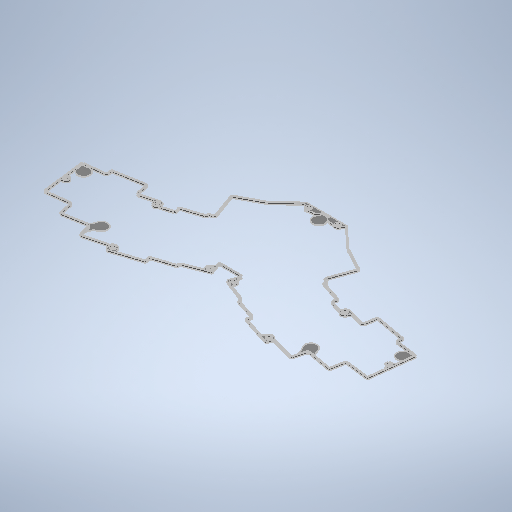
# Autodesk Inventor part: Hephaestus38v2 Case Bottom
Saved by Autodesk Inventor 2025 (Build 290162000, 162)
## iProperties
Created: 2025-11-22
Part Number: Hephaestus38v2 Case Bottom
Material: Generic
Document SubType Name: Modeling
Designer: User
Density: 1 g/cm^3
Appearance: Smooth - Black
Author: User
Autodesk Inventor part; units mm, degrees
(part 1 of 2)
ref_plane "YZ Plane" through (0, 0, 0) normal (1, 0, 0) x (0, 1, 0)
ref_plane "XZ Plane" through (0, 0, 0) normal (0, 1, 0) x (-1, 0, 0)
ref_plane "XY Plane" through (0, 0, 0) normal (0, 0, 1) x (1, 0, 0)
sketch "Sketch1" plane through (0, 0, 0) normal (0, 1, 0) x (-1, 0, 0)
  line L0 (-4.3858, 37.0574) -> (-22.4739, 44.0008)
  circle A0 centre (-7.0476, 34.7035) radius 1.1
  arc A1 (9.4036, 37.0574) -> (8.8284, 35.7654) centre (9.762, 36.1238) ccw
  line L1 (8.8284, 35.7654) -> (11.5745, 28.6116)
  arc A2 (10.6409, 27.2532) -> (11.5745, 28.6116) centre (10.641, 28.2531) ccw
  line L2 (10.6409, 27.2532) -> (-5.6231, 27.2532)
  arc A3 (-6.5567, 28.6116) -> (-5.6231, 27.2532) centre (-5.623, 28.2533) ccw
  line L3 (-6.5567, 28.6116) -> (-3.8105, 35.7654)
  arc A4 (-3.8105, 35.7654) -> (-4.3858, 37.0574) centre (-4.744, 36.1239) ccw
  line L4 (-4.3858, 37.0574) -> (-22.4739, 44.0008)
  arc A5 (-23.0666, 45.2434) -> (-22.4739, 44.0008) centre (-22.1155, 44.9344) ccw
  line L5 (-23.0666, 45.2434) -> (-22.9423, 45.6258)
  arc A6 (-22.9423, 45.6258) -> (-23.5844, 46.8859) centre (-23.8933, 45.9349) ccw
  circle A7 centre (12.0655, 34.7035) radius 1.1
  line L6 (10.6409, 27.2532) -> (-5.6231, 27.2532)
  arc A8 (10.6409, 27.2532) -> (11.5745, 28.6116) centre (10.641, 28.2531) ccw
  line L7 (-6.5567, 28.6116) -> (-3.8105, 35.7654)
  arc A9 (-3.8105, 35.7654) -> (-4.3858, 37.0574) centre (-4.744, 36.1239) ccw
  line L8 (8.8284, 35.7654) -> (11.5745, 28.6116)
  line L9 (27.4917, 44.0008) -> (9.4036, 37.0574)
  arc A10 (27.4917, 44.0008) -> (28.0844, 45.2433) centre (27.1334, 44.9343) ccw
  line L10 (27.9602, 45.6258) -> (28.0844, 45.2433)
  arc A11 (28.6022, 46.8859) -> (27.9602, 45.6258) centre (28.9113, 45.9348) ccw
  line L11 (44.7702, 52.1391) -> (28.6022, 46.8859)
  arc A12 (9.4036, 37.0574) -> (8.8284, 35.7654) centre (9.762, 36.1238) ccw
  arc A13 (45.2817, 57.0369) -> (44.6397, 55.7769) centre (45.5908, 56.0858) ccw
  line L12 (44.6397, 55.7769) -> (45.4122, 53.3992)
  arc A14 (44.7702, 52.1391) -> (45.4122, 53.3992) centre (44.4612, 53.0901) ccw
  line L13 (44.7702, 52.1391) -> (28.6022, 46.8859)
  arc A15 (28.6022, 46.8859) -> (27.9602, 45.6258) centre (28.9113, 45.9348) ccw
  line L14 (27.9602, 45.6258) -> (28.0844, 45.2433)
  arc A16 (27.4917, 44.0008) -> (28.0844, 45.2433) centre (27.1334, 44.9343) ccw
  line L15 (27.4917, 44.0008) -> (9.4036, 37.0574)
  line L16 (-23.5844, 46.8859) -> (-39.7523, 52.1392)
  arc A17 (-40.3944, 53.3993) -> (-39.7523, 52.1392) centre (-39.4433, 53.0903) ccw
  line L17 (-40.3944, 53.3993) -> (-39.6218, 55.7769)
  arc A18 (-39.6218, 55.7769) -> (-40.2638, 57.037) centre (-40.5728, 56.086) ccw
  circle A19 centre (-63.5707, 60.8956) radius 1.1
  circle A20 centre (68.5886, 60.8955) radius 1.1
  line L18 (20.0076, -53.7302) -> (36.7848, -38.2361)
  circle A21 centre (14.7393, -51.2055) radius 1.1
  arc A22 (-14.9899, -53.7302) -> (-14.3114, -53.9956) centre (-14.3114, -52.9955) ccw
  line L19 (-14.3114, -53.9956) -> (19.3291, -53.9956)
  line L20 (56.4521, -26.7701) -> (49.3032, -6.9462)
  arc A23 (36.9938, -38.0878) -> (36.7848, -38.2361) centre (37.4628, -38.97) ccw
  arc A24 (19.3291, -53.9956) -> (20.0076, -53.7302) centre (19.3291, -52.9954) ccw
  line L21 (20.0076, -53.7302) -> (36.7848, -38.2361)
  line L22 (36.9938, -38.0878) -> (55.9808, -27.9922)
  arc A25 (55.9808, -27.9922) -> (56.4521, -26.7701) centre (55.5114, -27.1093) ccw
  arc A26 (36.9938, -38.0878) -> (36.7848, -38.2361) centre (37.4628, -38.97) ccw
  line L23 (36.9938, -38.0878) -> (55.9808, -27.9922)
  arc A27 (55.9808, -27.9922) -> (56.4521, -26.7701) centre (55.5114, -27.1093) ccw
  line L24 (56.4521, -26.7701) -> (49.3032, -6.9462)
  arc A28 (53.4637, -2.2357) -> (52.8392, -3.5451) centre (53.7728, -3.1867) ccw
  line L25 (53.1719, -4.4119) -> (52.8392, -3.5451)
  line L26 (49.8855, -5.6734) -> (53.1719, -4.4119)
  arc A29 (69.7006, 7.7716) -> (69.0586, 6.5115) centre (70.0096, 6.8206) ccw
  line L27 (69.8311, 4.1339) -> (69.0586, 6.5115)
  arc A30 (69.1891, 2.8738) -> (69.8311, 4.1339) centre (68.8803, 3.8248) ccw
  line L28 (53.4637, -2.2357) -> (69.1891, 2.8738)
  line L29 (69.7006, 7.7716) -> (77.7078, 10.3732)
  arc A31 (78.9827, 9.681) -> (77.7078, 10.3732) centre (78.0168, 9.4221) ccw
  arc A32 (49.8855, -5.6734) -> (49.3032, -6.9462) centre (50.2437, -6.6069) ccw
  circle A33 centre (-76.6637, 9.8152) radius 1.1
  circle A34 centre (-133.8477, 29.6046) radius 1.1
  circle A35 centre (138.8656, 29.6043) radius 1.1
  circle A36 centre (81.6815, 9.8151) radius 1.1
  circle A37 centre (12.0655, 34.7035) radius 1.1
  circle A38 centre (-9.7216, -51.2055) radius 1.1
  circle A39 centre (-9.7216, -51.2055) radius 1.1
  circle A40 centre (14.7393, -51.2055) radius 1.1
  line L30 (-14.3114, -53.9956) -> (19.3291, -53.9956)
  arc A41 (-14.9899, -53.7302) -> (-14.3114, -53.9956) centre (-14.3114, -52.9955) ccw
  line L31 (-31.7671, -38.236) -> (-14.9899, -53.7302)
  arc A42 (19.3291, -53.9956) -> (20.0076, -53.7302) centre (19.3291, -52.9954) ccw
  arc A43 (-31.7671, -38.236) -> (-31.9761, -38.0877) centre (-32.4462, -38.9715) ccw
  line L32 (-50.9631, -27.9922) -> (-31.9761, -38.0877)
  arc A44 (-44.2854, -6.9461) -> (-44.8677, -5.6733) centre (-45.2262, -6.6069) ccw
  arc A45 (-51.4343, -26.77) -> (-50.9631, -27.9922) centre (-50.4936, -27.1092) ccw
  line L33 (-44.2854, -6.9461) -> (-51.4343, -26.77)
  line L34 (-47.2205, -4.7701) -> (-44.8677, -5.6733)
  arc A46 (-47.7958, -3.4782) -> (-47.2205, -4.7701) centre (-46.8621, -3.8365) ccw
  line L35 (-47.4437, -2.5612) -> (-47.7958, -3.4782)
  line L36 (-64.1713, 2.8739) -> (-47.4437, -2.5612)
  line L37 (-64.0408, 6.5116) -> (-64.8134, 4.134)
  arc A47 (-64.0408, 6.5116) -> (-64.6829, 7.7717) centre (-64.9919, 6.8206) ccw
  arc A48 (-64.8134, 4.134) -> (-64.1713, 2.8739) centre (-63.8622, 3.825) ccw
  line L38 (-72.69, 10.3734) -> (-64.6829, 7.7717)
  arc A49 (-75.8938, 6.3463) -> (-74.669, 7.0534) centre (-75.635, 7.3122) ccw
  line L39 (-74.669, 7.0534) -> (-73.9649, 9.6812)
  arc A50 (-72.69, 10.3734) -> (-73.9649, 9.6812) centre (-72.999, 9.4222) ccw
  line L40 (-111.7079, 56.9853) -> (-113.4989, 46.8282)
  line L41 (-120.3501, 7.9735) -> (-120.8071, 5.3814)
  arc A51 (-120.3501, 7.9735) -> (-121.213, 9.1397) centre (-121.3349, 8.1472) ccw
  line L42 (-137.7648, 11.1721) -> (-121.213, 9.1397)
  arc A52 (-133.2069, 48.2933) -> (-134.3213, 47.4226) centre (-133.3287, 47.3007) ccw
  line L43 (-134.3213, 47.4226) -> (-138.6355, 12.2865)
  arc A53 (-138.6355, 12.2865) -> (-137.7648, 11.1721) centre (-137.6431, 12.1645) ccw
  arc A54 (-90.8984, 54.3314) -> (-89.7588, 55.0574) centre (-90.7247, 55.3162) ccw
  arc A55 (-114.6056, 46.0093) -> (-113.4989, 46.8282) centre (-114.4838, 47.0019) ccw
  arc A56 (-110.5495, 57.7965) -> (-111.7079, 56.9853) centre (-110.7232, 56.8118) ccw
  line L44 (-114.6056, 46.0093) -> (-133.2069, 48.2933)
  line L45 (-90.8984, 54.3314) -> (-110.5495, 57.7965)
  line L46 (-40.2638, 57.037) -> (-64.0403, 64.7624)
  circle A57 centre (-63.5707, 60.8956) radius 1.1
  arc A58 (-67.5003, 60.4163) -> (-66.2904, 61.0732) centre (-67.2415, 61.3823) ccw
  arc A59 (-64.0403, 64.7624) -> (-65.3003, 64.1204) centre (-64.3492, 63.8113) ccw
  line L47 (-65.3003, 64.1204) -> (-66.2904, 61.0732)
  line L48 (-91.3846, 10.4971) -> (-75.8938, 6.3463)
  arc A60 (-95.3758, -0.1183) -> (-94.2173, 0.6929) centre (-95.2021, 0.8665) ccw
  arc A61 (-91.3846, 10.4971) -> (-92.6283, 9.7048) centre (-91.6435, 9.5312) ccw
  line L49 (-94.2173, 0.6929) -> (-92.6283, 9.7048)
  arc A62 (-120.8071, 5.3814) -> (-119.996, 4.2229) centre (-119.8224, 5.2077) ccw
  line L50 (-119.996, 4.2229) -> (-95.3758, -0.1183)
  arc A63 (69.7006, 7.7716) -> (69.0586, 6.5115) centre (70.0096, 6.8206) ccw
  arc A64 (53.4637, -2.2357) -> (52.8392, -3.5451) centre (53.7728, -3.1867) ccw
  line L51 (53.1719, -4.4119) -> (52.8392, -3.5451)
  line L52 (49.8855, -5.6734) -> (53.1719, -4.4119)
  line L53 (69.8311, 4.1339) -> (69.0586, 6.5115)
  arc A65 (69.1891, 2.8738) -> (69.8311, 4.1339) centre (68.8803, 3.8248) ccw
  line L54 (53.4637, -2.2357) -> (69.1891, 2.8738)
  line L55 (69.7006, 7.7716) -> (77.7078, 10.3732)
  arc A66 (49.8855, -5.6734) -> (49.3032, -6.9462) centre (50.2437, -6.6069) ccw
  line L56 (69.0581, 64.7623) -> (45.2817, 57.0369)
  arc A67 (70.3182, 64.1203) -> (69.0581, 64.7623) centre (69.3671, 63.8112) ccw
  arc A68 (71.3083, 61.0731) -> (72.5182, 60.4162) centre (72.2593, 61.3821) ccw
  line L57 (90.98, 65.363) -> (72.5182, 60.4162)
  arc A69 (92.2048, 64.6558) -> (90.98, 65.363) centre (91.2388, 64.397) ccw
  arc A70 (94.7767, 55.0573) -> (95.9163, 54.3313) centre (95.7426, 55.3161) ccw
  line L58 (94.7767, 55.0573) -> (92.2048, 64.6558)
  line L59 (71.3083, 61.0731) -> (70.3182, 64.1203)
  arc A71 (142.7826, 11.1718) -> (143.6533, 12.2863) centre (142.6606, 12.1645) ccw
  line L60 (78.9827, 9.681) -> (79.6868, 7.0532)
  arc A72 (79.6868, 7.0532) -> (80.9116, 6.3461) centre (80.6528, 7.3122) ccw
  line L61 (80.9116, 6.3461) -> (96.4024, 10.4969)
  arc A73 (97.6461, 9.7046) -> (96.4024, 10.4969) centre (96.6613, 9.531) ccw
  line L62 (97.6461, 9.7046) -> (99.2351, 0.6927)
  arc A74 (99.2351, 0.6927) -> (100.3935, -0.1185) centre (100.2199, 0.8664) ccw
  line L63 (100.3935, -0.1185) -> (125.0138, 4.2228)
  arc A75 (126.2308, 9.1395) -> (125.3678, 7.9733) centre (126.3526, 8.147) ccw
  arc A76 (125.0138, 4.2228) -> (125.8249, 5.3812) centre (124.8401, 5.2075) ccw
  line L64 (125.8249, 5.3812) -> (125.3678, 7.9733)
  line L65 (115.5673, 57.7963) -> (95.9163, 54.3313)
  arc A77 (116.7258, 56.9851) -> (115.5673, 57.7963) centre (115.7409, 56.8114) ccw
  line L66 (118.5167, 46.828) -> (116.7258, 56.9851)
  arc A78 (118.5167, 46.828) -> (119.6234, 46.0091) centre (119.5015, 47.0016) ccw
  arc A79 (139.3392, 47.4224) -> (138.2247, 48.2931) centre (138.3466, 47.3005) ccw
  line L67 (126.2308, 9.1395) -> (142.7826, 11.1718)
  line L68 (143.6533, 12.2863) -> (139.3392, 47.4224)
  arc A80 (142.7826, 11.1718) -> (143.6533, 12.2863) centre (142.6606, 12.1645) ccw
  line L69 (138.2247, 48.2931) -> (119.6234, 46.0091)
  circle A81 centre (68.5886, 60.8955) radius 1.1
  circle A82 centre (-7.0476, 34.7035) radius 1.1
  arc A83 (-31.7671, -38.236) -> (-31.9761, -38.0877) centre (-32.4462, -38.9715) ccw
  line L70 (-50.9631, -27.9922) -> (-31.9761, -38.0877)
  arc A84 (-51.4343, -26.77) -> (-50.9631, -27.9922) centre (-50.4936, -27.1092) ccw
  line L71 (-44.2854, -6.9461) -> (-51.4343, -26.77)
  arc A85 (-44.2854, -6.9461) -> (-44.8677, -5.6733) centre (-45.2262, -6.6069) ccw
  line L72 (-47.2205, -4.7701) -> (-44.8677, -5.6733)
  arc A86 (-47.7958, -3.4782) -> (-47.2205, -4.7701) centre (-46.8621, -3.8365) ccw
  line L73 (-47.4437, -2.5612) -> (-47.7958, -3.4782)
  circle A87 centre (-133.8477, 29.6046) radius 1.1
  line L74 (-31.7671, -38.236) -> (-14.9899, -53.7302)
  circle A88 centre (-76.6637, 9.8152) radius 1.1
  line L75 (-23.0666, 45.2434) -> (-22.9423, 45.6258)
  arc A89 (-23.0666, 45.2434) -> (-22.4739, 44.0008) centre (-22.1155, 44.9344) ccw
  arc A90 (-22.9423, 45.6258) -> (-23.5844, 46.8859) centre (-23.8933, 45.9349) ccw
  line L76 (-23.5844, 46.8859) -> (-39.7523, 52.1392)
  arc A91 (-39.6218, 55.7769) -> (-40.2638, 57.037) centre (-40.5728, 56.086) ccw
  line L77 (-40.3944, 53.3993) -> (-39.6218, 55.7769)
  arc A92 (-40.3944, 53.3993) -> (-39.7523, 52.1392) centre (-39.4433, 53.0903) ccw
  arc A93 (-6.5567, 28.6116) -> (-5.6231, 27.2532) centre (-5.623, 28.2533) ccw
  line L78 (-40.2638, 57.037) -> (-64.0403, 64.7624)
  arc A94 (-64.0403, 64.7624) -> (-65.3003, 64.1204) centre (-64.3492, 63.8113) ccw
  line L79 (-65.3003, 64.1204) -> (-66.2904, 61.0732)
  arc A95 (-67.5003, 60.4163) -> (-66.2904, 61.0732) centre (-67.2415, 61.3823) ccw
  arc A96 (94.7767, 55.0573) -> (95.9163, 54.3313) centre (95.7426, 55.3161) ccw
  circle A97 centre (81.6815, 9.8151) radius 1.1
  line L80 (100.3935, -0.1185) -> (125.0138, 4.2228)
  arc A98 (125.0138, 4.2228) -> (125.8249, 5.3812) centre (124.8401, 5.2075) ccw
  arc A99 (99.2351, 0.6927) -> (100.3935, -0.1185) centre (100.2199, 0.8664) ccw
  arc A100 (78.9827, 9.681) -> (77.7078, 10.3732) centre (78.0168, 9.4221) ccw
  line L81 (78.9827, 9.681) -> (79.6868, 7.0532)
  arc A101 (79.6868, 7.0532) -> (80.9116, 6.3461) centre (80.6528, 7.3122) ccw
  line L82 (80.9116, 6.3461) -> (96.4024, 10.4969)
  arc A102 (97.6461, 9.7046) -> (96.4024, 10.4969) centre (96.6613, 9.531) ccw
  line L83 (125.8249, 5.3812) -> (125.3678, 7.9733)
  arc A103 (126.2308, 9.1395) -> (125.3678, 7.9733) centre (126.3526, 8.147) ccw
  line L84 (97.6461, 9.7046) -> (99.2351, 0.6927)
  circle A104 centre (138.8656, 29.6043) radius 1.1
  arc A105 (118.5167, 46.828) -> (119.6234, 46.0091) centre (119.5015, 47.0016) ccw
  line L85 (138.2247, 48.2931) -> (119.6234, 46.0091)
  line L86 (126.2308, 9.1395) -> (142.7826, 11.1718)
  arc A106 (139.3392, 47.4224) -> (138.2247, 48.2931) centre (138.3466, 47.3005) ccw
  line L87 (143.6533, 12.2863) -> (139.3392, 47.4224)
  arc A107 (71.3083, 61.0731) -> (72.5182, 60.4162) centre (72.2593, 61.3821) ccw
  line L88 (90.98, 65.363) -> (72.5182, 60.4162)
  arc A108 (92.2048, 64.6558) -> (90.98, 65.363) centre (91.2388, 64.397) ccw
  line L89 (94.7767, 55.0573) -> (92.2048, 64.6558)
  line L90 (115.5673, 57.7963) -> (95.9163, 54.3313)
  arc A109 (116.7258, 56.9851) -> (115.5673, 57.7963) centre (115.7409, 56.8114) ccw
  line L91 (118.5167, 46.828) -> (116.7258, 56.9851)
  arc A110 (44.7702, 52.1391) -> (45.4122, 53.3992) centre (44.4612, 53.0901) ccw
  line L92 (44.6397, 55.7769) -> (45.4122, 53.3992)
  arc A111 (45.2817, 57.0369) -> (44.6397, 55.7769) centre (45.5908, 56.0858) ccw
  line L93 (69.0581, 64.7623) -> (45.2817, 57.0369)
  line L94 (71.3083, 61.0731) -> (70.3182, 64.1203)
  arc A112 (70.3182, 64.1203) -> (69.0581, 64.7623) centre (69.3671, 63.8112) ccw
  line L95 (-72.69, 10.3734) -> (-64.6829, 7.7717)
  arc A113 (-72.69, 10.3734) -> (-73.9649, 9.6812) centre (-72.999, 9.4222) ccw
  line L96 (-74.669, 7.0534) -> (-73.9649, 9.6812)
  arc A114 (-75.8938, 6.3463) -> (-74.669, 7.0534) centre (-75.635, 7.3122) ccw
  line L97 (-91.3846, 10.4971) -> (-75.8938, 6.3463)
  arc A115 (-91.3846, 10.4971) -> (-92.6283, 9.7048) centre (-91.6435, 9.5312) ccw
  line L98 (-94.2173, 0.6929) -> (-92.6283, 9.7048)
  arc A116 (-138.6355, 12.2865) -> (-137.7648, 11.1721) centre (-137.6431, 12.1645) ccw
  line L99 (-137.7648, 11.1721) -> (-121.213, 9.1397)
  arc A117 (-120.3501, 7.9735) -> (-121.213, 9.1397) centre (-121.3349, 8.1472) ccw
  line L100 (-120.3501, 7.9735) -> (-120.8071, 5.3814)
  arc A118 (-120.8071, 5.3814) -> (-119.996, 4.2229) centre (-119.8224, 5.2077) ccw
  line L101 (-119.996, 4.2229) -> (-95.3758, -0.1183)
  arc A119 (-133.2069, 48.2933) -> (-134.3213, 47.4226) centre (-133.3287, 47.3007) ccw
  arc A120 (-114.6056, 46.0093) -> (-113.4989, 46.8282) centre (-114.4838, 47.0019) ccw
  line L102 (-114.6056, 46.0093) -> (-133.2069, 48.2933)
  line L103 (-67.5003, 60.4163) -> (-85.9621, 65.3631)
  line L104 (-67.5003, 60.4163) -> (-85.9621, 65.3631)
  line L105 (-64.1713, 2.8739) -> (-47.4437, -2.5612)
  arc A121 (-64.8134, 4.134) -> (-64.1713, 2.8739) centre (-63.8622, 3.825) ccw
  line L106 (-64.0408, 6.5116) -> (-64.8134, 4.134)
  arc A122 (-64.0408, 6.5116) -> (-64.6829, 7.7717) centre (-64.9919, 6.8206) ccw
  arc A123 (-95.3758, -0.1183) -> (-94.2173, 0.6929) centre (-95.2021, 0.8665) ccw
  line L107 (-90.8984, 54.3314) -> (-110.5495, 57.7965)
  line L108 (-111.7079, 56.9853) -> (-113.4989, 46.8282)
  arc A124 (-85.9621, 65.3631) -> (-87.1869, 64.656) centre (-86.2209, 64.3972) ccw
  arc A125 (-85.9621, 65.3631) -> (-87.1869, 64.656) centre (-86.2209, 64.3972) ccw
  line L109 (-87.1869, 64.656) -> (-89.7588, 55.0574)
  line L110 (-87.1869, 64.656) -> (-89.7588, 55.0574)
  arc A126 (-90.8984, 54.3314) -> (-89.7588, 55.0574) centre (-90.7247, 55.3162) ccw
  arc A127 (-110.5495, 57.7965) -> (-111.7079, 56.9853) centre (-110.7232, 56.8118) ccw
  line L111 (-134.3213, 47.4226) -> (-138.6355, 12.2865)
  constraints: 224 end point, 216 point on circle, 128 centre point, 2 horizontal, 476 other
extrude "Extrusion1" add sketch "Sketch1" along normal blind 1.6
sketch "Sketch2" plane through (0, 1.6, 0) normal (0, 1, 0) x (1, 0, 0)
  arc A0 (90.8984, -54.3314) -> (89.7588, -55.0574) centre (90.7247, -55.3162) ccw projected
  line L0 (90.8984, -54.3314) -> (110.5495, -57.7965) projected
  arc A1 (110.5495, -57.7965) -> (111.7079, -56.9853) centre (110.7232, -56.8118) ccw projected
  line L1 (111.7079, -56.9853) -> (113.4989, -46.8282) projected
  arc A2 (114.6056, -46.0093) -> (113.4989, -46.8282) centre (114.4838, -47.0019) ccw projected
  line L2 (114.6056, -46.0093) -> (133.2069, -48.2933) projected
  arc A3 (133.2069, -48.2933) -> (134.3213, -47.4226) centre (133.3287, -47.3007) ccw projected
  line L3 (134.3213, -47.4226) -> (138.6355, -12.2865) projected
  arc A4 (138.6355, -12.2865) -> (137.7648, -11.1721) centre (137.6431, -12.1645) ccw projected
  line L4 (137.7648, -11.1721) -> (121.213, -9.1397) projected
  arc A5 (120.3501, -7.9735) -> (121.213, -9.1397) centre (121.3349, -8.1472) ccw projected
  line L5 (120.3501, -7.9735) -> (120.8071, -5.3814) projected
  arc A6 (120.8071, -5.3814) -> (119.996, -4.2229) centre (119.8224, -5.2077) ccw projected
  line L6 (119.996, -4.2229) -> (95.3758, 0.1183) projected
  arc A7 (95.3758, 0.1183) -> (94.2173, -0.6929) centre (95.2021, -0.8665) ccw projected
  line L7 (94.2173, -0.6929) -> (92.6283, -9.7048) projected
  arc A8 (91.3846, -10.4971) -> (92.6283, -9.7048) centre (91.6435, -9.5312) ccw projected
  line L8 (91.3846, -10.4971) -> (75.8938, -6.3463) projected
  arc A9 (75.8938, -6.3463) -> (74.669, -7.0534) centre (75.635, -7.3122) ccw projected
  line L9 (74.669, -7.0534) -> (73.9649, -9.6812) projected
  arc A10 (72.69, -10.3734) -> (73.9649, -9.6812) centre (72.999, -9.4222) ccw projected
  line L10 (72.69, -10.3734) -> (64.6829, -7.7717) projected
  arc A11 (64.0408, -6.5116) -> (64.6829, -7.7717) centre (64.9919, -6.8206) ccw projected
  line L11 (64.0408, -6.5116) -> (64.8134, -4.134) projected
  arc A12 (64.8134, -4.134) -> (64.1713, -2.8739) centre (63.8622, -3.825) ccw projected
  line L12 (64.1713, -2.8739) -> (47.4437, 2.5612) projected
  line L13 (47.4437, 2.5612) -> (47.7958, 3.4782) projected
  arc A13 (47.7958, 3.4782) -> (47.2205, 4.7701) centre (46.8621, 3.8365) ccw projected
  line L14 (47.2205, 4.7701) -> (44.8677, 5.6733) projected
  arc A14 (44.2854, 6.9461) -> (44.8677, 5.6733) centre (45.2262, 6.6069) ccw projected
  line L15 (44.2854, 6.9461) -> (51.4343, 26.77) projected
  arc A15 (51.4343, 26.77) -> (50.9631, 27.9922) centre (50.4936, 27.1092) ccw projected
  line L16 (50.9631, 27.9922) -> (31.9761, 38.0877) projected
  arc A16 (31.7671, 38.236) -> (31.9761, 38.0877) centre (32.4462, 38.9715) ccw projected
  line L17 (31.7671, 38.236) -> (14.9899, 53.7302) projected
  arc A17 (14.9899, 53.7302) -> (14.3114, 53.9956) centre (14.3114, 52.9955) ccw projected
  line L18 (14.3114, 53.9956) -> (-19.3291, 53.9956) projected
  arc A18 (-19.3291, 53.9956) -> (-20.0076, 53.7302) centre (-19.3291, 52.9954) ccw projected
  line L19 (-20.0076, 53.7302) -> (-36.7848, 38.2361) projected
  arc A19 (-36.9938, 38.0878) -> (-36.7848, 38.2361) centre (-37.4628, 38.97) ccw projected
  line L20 (-36.9938, 38.0878) -> (-55.9808, 27.9922) projected
  arc A20 (-55.9808, 27.9922) -> (-56.4521, 26.7701) centre (-55.5114, 27.1093) ccw projected
  line L21 (-56.4521, 26.7701) -> (-49.3032, 6.9462) projected
  arc A21 (-49.8855, 5.6734) -> (-49.3032, 6.9462) centre (-50.2437, 6.6069) ccw projected
  line L22 (-49.8855, 5.6734) -> (-53.1719, 4.4119) projected
  line L23 (-53.1719, 4.4119) -> (-52.8392, 3.5451) projected
  arc A22 (-53.4637, 2.2357) -> (-52.8392, 3.5451) centre (-53.7728, 3.1867) ccw projected
  line L24 (-53.4637, 2.2357) -> (-69.1891, -2.8738) projected
  arc A23 (-69.1891, -2.8738) -> (-69.8311, -4.1339) centre (-68.8803, -3.8248) ccw projected
  line L25 (-69.8311, -4.1339) -> (-69.0586, -6.5115) projected
  arc A24 (-69.7006, -7.7716) -> (-69.0586, -6.5115) centre (-70.0096, -6.8206) ccw projected
  line L26 (-69.7006, -7.7716) -> (-77.7078, -10.3732) projected
  arc A25 (-78.9827, -9.681) -> (-77.7078, -10.3732) centre (-78.0168, -9.4221) ccw projected
  line L27 (-78.9827, -9.681) -> (-79.6868, -7.0532) projected
  arc A26 (-79.6868, -7.0532) -> (-80.9116, -6.3461) centre (-80.6528, -7.3122) ccw projected
  line L28 (-80.9116, -6.3461) -> (-96.4024, -10.4969) projected
  arc A27 (-97.6461, -9.7046) -> (-96.4024, -10.4969) centre (-96.6613, -9.531) ccw projected
  line L29 (-97.6461, -9.7046) -> (-99.2351, -0.6927) projected
  arc A28 (-99.2351, -0.6927) -> (-100.3935, 0.1185) centre (-100.2199, -0.8664) ccw projected
  line L30 (-100.3935, 0.1185) -> (-125.0138, -4.2228) projected
  arc A29 (-125.0138, -4.2228) -> (-125.8249, -5.3812) centre (-124.8401, -5.2075) ccw projected
  line L31 (-125.8249, -5.3812) -> (-125.3678, -7.9733) projected
  arc A30 (-126.2308, -9.1395) -> (-125.3678, -7.9733) centre (-126.3526, -8.147) ccw projected
  line L32 (-126.2308, -9.1395) -> (-142.7826, -11.1718) projected
  arc A31 (-142.7826, -11.1718) -> (-143.6533, -12.2863) centre (-142.6606, -12.1645) ccw projected
  line L33 (-143.6533, -12.2863) -> (-139.3392, -47.4224) projected
  arc A32 (-139.3392, -47.4224) -> (-138.2247, -48.2931) centre (-138.3466, -47.3005) ccw projected
  line L34 (-138.2247, -48.2931) -> (-119.6234, -46.0091) projected
  arc A33 (-118.5167, -46.828) -> (-119.6234, -46.0091) centre (-119.5015, -47.0016) ccw projected
  line L35 (-118.5167, -46.828) -> (-116.7258, -56.9851) projected
  arc A34 (-116.7258, -56.9851) -> (-115.5673, -57.7963) centre (-115.7409, -56.8114) ccw projected
  line L36 (-115.5673, -57.7963) -> (-95.9163, -54.3313) projected
  arc A35 (-94.7767, -55.0573) -> (-95.9163, -54.3313) centre (-95.7426, -55.3161) ccw projected
  line L37 (-94.7767, -55.0573) -> (-92.2048, -64.6558) projected
  arc A36 (-92.2048, -64.6558) -> (-90.98, -65.363) centre (-91.2388, -64.397) ccw projected
  line L38 (-90.98, -65.363) -> (-72.5182, -60.4162) projected
  arc A37 (-71.3083, -61.0731) -> (-72.5182, -60.4162) centre (-72.2593, -61.3821) ccw projected
  line L39 (-71.3083, -61.0731) -> (-70.3182, -64.1203) projected
  arc A38 (-70.3182, -64.1203) -> (-69.0581, -64.7623) centre (-69.3671, -63.8112) ccw projected
  line L40 (-69.0581, -64.7623) -> (-45.2817, -57.0369) projected
  arc A39 (-45.2817, -57.0369) -> (-44.6397, -55.7769) centre (-45.5908, -56.0858) ccw projected
  line L41 (-44.6397, -55.7769) -> (-45.4122, -53.3992) projected
  arc A40 (-44.7702, -52.1391) -> (-45.4122, -53.3992) centre (-44.4612, -53.0901) ccw projected
  line L42 (-44.7702, -52.1391) -> (-28.6022, -46.8859) projected
  arc A41 (-28.6022, -46.8859) -> (-27.9602, -45.6258) centre (-28.9113, -45.9348) ccw projected
  line L43 (-27.9602, -45.6258) -> (-28.0844, -45.2433) projected
  arc A42 (-27.4917, -44.0008) -> (-28.0844, -45.2433) centre (-27.1334, -44.9343) ccw projected
  line L44 (-27.4917, -44.0008) -> (-9.4036, -37.0574) projected
  arc A43 (-9.4036, -37.0574) -> (-8.8284, -35.7654) centre (-9.762, -36.1238) ccw projected
  line L45 (-8.8284, -35.7654) -> (-11.5745, -28.6116) projected
  arc A44 (-10.6409, -27.2532) -> (-11.5745, -28.6116) centre (-10.641, -28.2531) ccw projected
  line L46 (-10.6409, -27.2532) -> (5.6231, -27.2532) projected
  arc A45 (6.5567, -28.6116) -> (5.6231, -27.2532) centre (5.623, -28.2533) ccw projected
  line L47 (6.5567, -28.6116) -> (3.8105, -35.7654) projected
  arc A46 (3.8105, -35.7654) -> (4.3858, -37.0574) centre (4.744, -36.1239) ccw projected
  line L48 (4.3858, -37.0574) -> (22.4739, -44.0008) projected
  arc A47 (23.0666, -45.2434) -> (22.4739, -44.0008) centre (22.1155, -44.9344) ccw projected
  line L49 (23.0666, -45.2434) -> (22.9423, -45.6258) projected
  arc A48 (22.9423, -45.6258) -> (23.5844, -46.8859) centre (23.8933, -45.9349) ccw projected
  line L50 (23.5844, -46.8859) -> (39.7523, -52.1392) projected
  arc A49 (40.3944, -53.3993) -> (39.7523, -52.1392) centre (39.4433, -53.0903) ccw projected
  line L51 (40.3944, -53.3993) -> (39.6218, -55.7769) projected
  arc A50 (39.6218, -55.7769) -> (40.2638, -57.037) centre (40.5728, -56.086) ccw projected
  line L52 (40.2638, -57.037) -> (64.0403, -64.7624) projected
  arc A51 (64.0403, -64.7624) -> (65.3003, -64.1204) centre (64.3492, -63.8113) ccw projected
  line L53 (65.3003, -64.1204) -> (66.2904, -61.0732) projected
  arc A52 (67.5003, -60.4163) -> (66.2904, -61.0732) centre (67.2415, -61.3823) ccw projected
  line L54 (67.5003, -60.4163) -> (85.9621, -65.3631) projected
  arc A53 (85.9621, -65.3631) -> (87.1869, -64.656) centre (86.2209, -64.3972) ccw projected
  line L55 (87.1869, -64.656) -> (89.7588, -55.0574) projected
  circle A54 centre (9.7216, 51.2055) radius 1.1 projected
  circle A55 centre (-138.8656, -29.6043) radius 1.1 projected
  circle A56 centre (76.6637, -9.8152) radius 1.1 projected
  circle A57 centre (-14.7393, 51.2055) radius 1.1 projected
  circle A58 centre (-68.5886, -60.8955) radius 1.1 projected
  circle A59 centre (63.5707, -60.8956) radius 1.1 projected
  circle A60 centre (-12.0655, -34.7035) radius 1.1 projected
  circle A61 centre (7.0476, -34.7035) radius 1.1 projected
  circle A62 centre (133.8477, -29.6046) radius 1.1 projected
  circle A63 centre (-81.6815, -9.8151) radius 1.1 projected
  circle A64 centre (-14.7393, 51.2055) radius 2.25
  circle A65 centre (9.7216, 51.2055) radius 2.25
  circle A66 centre (76.6637, -9.8152) radius 2.25
  circle A67 centre (133.8477, -29.6046) radius 2.25
  circle A68 centre (63.5707, -60.8956) radius 2.25
  circle A69 centre (7.0476, -34.7035) radius 2.25
  circle A70 centre (-12.0655, -34.7035) radius 2.25
  circle A71 centre (-68.5886, -60.8955) radius 2.25
  circle A72 centre (-138.8656, -29.6043) radius 2.25
  circle A73 centre (-81.6815, -9.8151) radius 2.25
  point P0 (0, 0)
  dimension "d2" = 4.5
  constraints: 10 centre point, 10 coincident, 9 equal radius
  measures "d2" diameter of A64
extrude "Extrusion2" cut sketch "Sketch2" against normal blind 1.2 contours A64 | A65 | A66 | A67 | A68 | A69 | A70 | A71 | A72 | A73
sketch "Sketch3" plane through (0, 1.6, 0) normal (0, 1, 0) x (1, 0, 0)
  circle A0 centre (76.6637, -9.8152) radius 1.6 projected
  arc A1 (74.0258, -11.5396) -> (72.3618, -10.2668) centre (71.388, -13.264) ccw projected
  arc A2 (74.0258, -11.5396) -> (79.7078, -10.6309) centre (76.6637, -9.8152) ccw projected
  arc A3 (83.5675, -8.4025) -> (79.7078, -10.6309) centre (82.7519, -11.4465) ccw projected
  line L0 (75.8938, -6.3463) -> (83.5675, -8.4025) projected
  arc A4 (75.8938, -6.3463) -> (74.669, -7.0534) centre (75.635, -7.3122) ccw projected
  line L1 (73.9649, -9.6812) -> (74.669, -7.0534) projected
  arc A5 (72.69, -10.3734) -> (73.9649, -9.6812) centre (72.999, -9.4222) ccw projected
  line L2 (72.3618, -10.2668) -> (72.69, -10.3734) projected
  arc A6 (134.1697, -26.9828) -> (137.1134, -24.6829) centre (134.4916, -24.3609) ccw projected
  arc A7 (134.1697, -26.9828) -> (133.5258, -32.2264) centre (133.8477, -29.6046) ccw projected
  arc A8 (135.8257, -35.1702) -> (133.5258, -32.2264) centre (133.2039, -34.8482) ccw projected
  line L3 (137.1134, -24.6829) -> (135.8257, -35.1702) projected
  circle A9 centre (133.8477, -29.6046) radius 1.6 projected
  circle A10 centre (63.5707, -60.8956) radius 1.6 projected
  arc A11 (66.6239, -59.119) -> (68.7628, -60.7546) centre (69.6771, -57.3425) ccw projected
  arc A12 (66.6239, -59.119) -> (60.2111, -59.804) centre (63.5707, -60.8956) ccw projected
  arc A13 (55.7599, -62.072) -> (60.2111, -59.804) centre (56.8515, -58.7124) ccw projected
  line L4 (64.0403, -64.7624) -> (55.7599, -62.072) projected
  arc A14 (64.0403, -64.7624) -> (65.3003, -64.1204) centre (64.3492, -63.8113) ccw projected
  line L5 (66.2904, -61.0732) -> (65.3003, -64.1204) projected
  arc A15 (67.5003, -60.4163) -> (66.2904, -61.0732) centre (67.2415, -61.3823) ccw projected
  line L6 (68.7628, -60.7546) -> (67.5003, -60.4163) projected
  circle A16 centre (7.0476, -34.7035) radius 1.6 projected
  arc A17 (9.9898, -35.8329) -> (11.8026, -39.9045) centre (12.932, -36.9623) ccw projected
  arc A18 (9.9898, -35.8329) -> (8.0291, -31.7087) centre (7.0476, -34.7035) ccw projected
  arc A19 (6.5567, -28.6116) -> (8.0291, -31.7087) centre (8.7661, -29.4597) ccw projected
  line L7 (3.8105, -35.7654) -> (6.5567, -28.6116) projected
  arc A20 (3.8105, -35.7654) -> (4.3858, -37.0574) centre (4.744, -36.1239) ccw projected
  line L8 (11.8026, -39.9045) -> (4.3858, -37.0574) projected
  circle A21 centre (-12.0655, -34.7035) radius 1.6 projected
  arc A22 (-16.8204, -39.9044) -> (-15.0076, -35.8329) centre (-17.9498, -36.9623) ccw projected
  line L9 (-9.4036, -37.0574) -> (-16.8204, -39.9044) projected
  arc A23 (-9.4036, -37.0574) -> (-8.8284, -35.7654) centre (-9.762, -36.1238) ccw projected
  line L10 (-11.5745, -28.6116) -> (-8.8284, -35.7654) projected
  arc A24 (-13.0469, -31.7087) -> (-11.5745, -28.6116) centre (-13.784, -29.4597) ccw projected
  arc A25 (-13.0469, -31.7087) -> (-15.0076, -35.8329) centre (-12.0655, -34.7035) ccw projected
  arc A26 (-73.7808, -60.7545) -> (-71.6418, -59.1189) centre (-74.695, -57.3423) ccw projected
  line L11 (-72.5182, -60.4162) -> (-73.7808, -60.7545) projected
  arc A27 (-71.3083, -61.0731) -> (-72.5182, -60.4162) centre (-72.2593, -61.3821) ccw projected
  line L12 (-70.3182, -64.1203) -> (-71.3083, -61.0731) projected
  arc A28 (-70.3182, -64.1203) -> (-69.0581, -64.7623) centre (-69.3671, -63.8112) ccw projected
  line L13 (-60.7778, -62.0719) -> (-69.0581, -64.7623) projected
  arc A29 (-65.229, -59.8039) -> (-60.7778, -62.0719) centre (-61.8694, -58.7123) ccw projected
  arc A30 (-65.229, -59.8039) -> (-71.6418, -59.1189) centre (-68.5886, -60.8955) ccw projected
  circle A31 centre (-68.5886, -60.8955) radius 1.6 projected
  circle A32 centre (-138.8656, -29.6043) radius 1.6 projected
  arc A33 (-142.1312, -24.6826) -> (-139.1875, -26.9825) centre (-139.5094, -24.3607) ccw projected
  line L14 (-140.8436, -35.1699) -> (-142.1312, -24.6826) projected
  arc A34 (-138.5437, -32.2262) -> (-140.8436, -35.1699) centre (-138.2217, -34.848) ccw projected
  arc A35 (-138.5437, -32.2262) -> (-139.1875, -26.9825) centre (-138.8656, -29.6043) ccw projected
  circle A36 centre (-14.7393, 51.2055) radius 1.6 projected
  arc A37 (-17.4405, 50.507) -> (-22.0347, 51.8582) centre (-20.1417, 49.8085) ccw projected
  arc A38 (-17.4405, 50.507) -> (-13.7066, 48.6137) centre (-14.7393, 51.2055) ccw projected
  arc A39 (-5.6088, 48.7956) -> (-13.7066, 48.6137) centre (-9.4136, 37.8395) ccw projected
  line L15 (-5.6088, 48.7956) -> (-5.6088, 52.7956) projected
  arc A40 (-5.6088, 52.7956) -> (-6.0088, 53.9956) centre (-7.6088, 52.7956) ccw projected
  line L16 (-19.3291, 53.9956) -> (-6.0088, 53.9956) projected
  arc A41 (-19.3291, 53.9956) -> (-20.0076, 53.7302) centre (-19.3291, 52.9954) ccw projected
  line L17 (-22.0347, 51.8582) -> (-20.0076, 53.7302) projected
  arc A42 (8.6889, 48.6136) -> (0.5912, 48.7956) centre (4.3959, 37.8394) ccw projected
  arc A43 (8.6889, 48.6136) -> (12.4228, 50.507) centre (9.7216, 51.2055) ccw projected
  arc A44 (17.017, 51.8581) -> (12.4228, 50.507) centre (15.124, 49.8084) ccw projected
  line L18 (14.9899, 53.7302) -> (17.017, 51.8581) projected
  arc A45 (14.9899, 53.7302) -> (14.3114, 53.9956) centre (14.3114, 52.9955) ccw projected
  line L19 (0.9912, 53.9956) -> (14.3114, 53.9956) projected
  arc A46 (0.9912, 53.9956) -> (0.5912, 52.7956) centre (2.5912, 52.7956) ccw projected
  line L20 (0.5912, 52.7956) -> (0.5912, 48.7956) projected
  circle A47 centre (9.7216, 51.2055) radius 1.6 projected
  circle A48 centre (63.5707, -60.8956) radius 2.25 projected
  circle A49 centre (-14.7393, 51.2055) radius 2.25 projected
  circle A50 centre (-68.5886, -60.8955) radius 2.25 projected
  circle A51 centre (9.7216, 51.2055) radius 2.25 projected
  circle A52 centre (7.0476, -34.7035) radius 2.25 projected
  circle A53 centre (133.8477, -29.6046) radius 2.25 projected
  circle A54 centre (-81.6815, -9.8151) radius 2.25 projected
  circle A55 centre (-138.8656, -29.6043) radius 2.25 projected
  circle A56 centre (76.6637, -9.8152) radius 2.25 projected
  circle A57 centre (-12.0655, -34.7035) radius 2.25 projected
  arc A58 (90.8984, -54.3314) -> (89.7588, -55.0574) centre (90.7247, -55.3162) ccw projected
  line L21 (90.8984, -54.3314) -> (110.5495, -57.7965) projected
  arc A59 (110.5495, -57.7965) -> (111.7079, -56.9853) centre (110.7232, -56.8118) ccw projected
  line L22 (111.7079, -56.9853) -> (113.4989, -46.8282) projected
  arc A60 (114.6056, -46.0093) -> (113.4989, -46.8282) centre (114.4838, -47.0019) ccw projected
  line L23 (114.6056, -46.0093) -> (133.2069, -48.2933) projected
  arc A61 (133.2069, -48.2933) -> (134.3213, -47.4226) centre (133.3287, -47.3007) ccw projected
  line L24 (134.3213, -47.4226) -> (138.6355, -12.2865) projected
  arc A62 (138.6355, -12.2865) -> (137.7648, -11.1721) centre (137.6431, -12.1645) ccw projected
  line L25 (137.7648, -11.1721) -> (121.213, -9.1397) projected
  arc A63 (120.3501, -7.9735) -> (121.213, -9.1397) centre (121.3349, -8.1472) ccw projected
  line L26 (120.3501, -7.9735) -> (120.8071, -5.3814) projected
  arc A64 (120.8071, -5.3814) -> (119.996, -4.2229) centre (119.8224, -5.2077) ccw projected
  line L27 (119.996, -4.2229) -> (95.3758, 0.1183) projected
  arc A65 (95.3758, 0.1183) -> (94.2173, -0.6929) centre (95.2021, -0.8665) ccw projected
  line L28 (94.2173, -0.6929) -> (92.6283, -9.7048) projected
  arc A66 (91.3846, -10.4971) -> (92.6283, -9.7048) centre (91.6435, -9.5312) ccw projected
  line L29 (91.3846, -10.4971) -> (75.8938, -6.3463) projected
  arc A67 (75.8938, -6.3463) -> (74.669, -7.0534) centre (75.635, -7.3122) ccw projected
  line L30 (74.669, -7.0534) -> (73.9649, -9.6812) projected
  arc A68 (72.69, -10.3734) -> (73.9649, -9.6812) centre (72.999, -9.4222) ccw projected
  line L31 (72.69, -10.3734) -> (64.6829, -7.7717) projected
  arc A69 (64.0408, -6.5116) -> (64.6829, -7.7717) centre (64.9919, -6.8206) ccw projected
  line L32 (64.0408, -6.5116) -> (64.8134, -4.134) projected
  arc A70 (64.8134, -4.134) -> (64.1713, -2.8739) centre (63.8622, -3.825) ccw projected
  line L33 (64.1713, -2.8739) -> (47.4437, 2.5612) projected
  line L34 (47.4437, 2.5612) -> (47.7958, 3.4782) projected
  arc A71 (47.7958, 3.4782) -> (47.2205, 4.7701) centre (46.8621, 3.8365) ccw projected
  line L35 (47.2205, 4.7701) -> (44.8677, 5.6733) projected
  arc A72 (44.2854, 6.9461) -> (44.8677, 5.6733) centre (45.2262, 6.6069) ccw projected
  line L36 (44.2854, 6.9461) -> (51.4343, 26.77) projected
  arc A73 (51.4343, 26.77) -> (50.9631, 27.9922) centre (50.4936, 27.1092) ccw projected
  line L37 (50.9631, 27.9922) -> (31.9761, 38.0877) projected
  arc A74 (31.7671, 38.236) -> (31.9761, 38.0877) centre (32.4462, 38.9715) ccw projected
  line L38 (31.7671, 38.236) -> (14.9899, 53.7302) projected
  arc A75 (14.9899, 53.7302) -> (14.3114, 53.9956) centre (14.3114, 52.9955) ccw projected
  line L39 (14.3114, 53.9956) -> (-19.3291, 53.9956) projected
  arc A76 (-19.3291, 53.9956) -> (-20.0076, 53.7302) centre (-19.3291, 52.9954) ccw projected
  line L40 (-20.0076, 53.7302) -> (-36.7848, 38.2361) projected
  arc A77 (-36.9938, 38.0878) -> (-36.7848, 38.2361) centre (-37.4628, 38.97) ccw projected
  line L41 (-36.9938, 38.0878) -> (-55.9808, 27.9922) projected
  arc A78 (-55.9808, 27.9922) -> (-56.4521, 26.7701) centre (-55.5114, 27.1093) ccw projected
  line L42 (-56.4521, 26.7701) -> (-49.3032, 6.9462) projected
  arc A79 (-49.8855, 5.6734) -> (-49.3032, 6.9462) centre (-50.2437, 6.6069) ccw projected
  line L43 (-49.8855, 5.6734) -> (-53.1719, 4.4119) projected
  line L44 (-53.1719, 4.4119) -> (-52.8392, 3.5451) projected
  arc A80 (-53.4637, 2.2357) -> (-52.8392, 3.5451) centre (-53.7728, 3.1867) ccw projected
  line L45 (-53.4637, 2.2357) -> (-69.1891, -2.8738) projected
  arc A81 (-69.1891, -2.8738) -> (-69.8311, -4.1339) centre (-68.8803, -3.8248) ccw projected
  line L46 (-69.8311, -4.1339) -> (-69.0586, -6.5115) projected
  arc A82 (-69.7006, -7.7716) -> (-69.0586, -6.5115) centre (-70.0096, -6.8206) ccw projected
  line L47 (-69.7006, -7.7716) -> (-77.7078, -10.3732) projected
  arc A83 (-78.9827, -9.681) -> (-77.7078, -10.3732) centre (-78.0168, -9.4221) ccw projected
  line L48 (-78.9827, -9.681) -> (-79.6868, -7.0532) projected
  arc A84 (-79.6868, -7.0532) -> (-80.9116, -6.3461) centre (-80.6528, -7.3122) ccw projected
  line L49 (-80.9116, -6.3461) -> (-96.4024, -10.4969) projected
  arc A85 (-97.6461, -9.7046) -> (-96.4024, -10.4969) centre (-96.6613, -9.531) ccw projected
  line L50 (-97.6461, -9.7046) -> (-99.2351, -0.6927) projected
  arc A86 (-99.2351, -0.6927) -> (-100.3935, 0.1185) centre (-100.2199, -0.8664) ccw projected
  line L51 (-100.3935, 0.1185) -> (-125.0138, -4.2228) projected
  arc A87 (-125.0138, -4.2228) -> (-125.8249, -5.3812) centre (-124.8401, -5.2075) ccw projected
  line L52 (-125.8249, -5.3812) -> (-125.3678, -7.9733) projected
  arc A88 (-126.2308, -9.1395) -> (-125.3678, -7.9733) centre (-126.3526, -8.147) ccw projected
  line L53 (-126.2308, -9.1395) -> (-142.7826, -11.1718) projected
  arc A89 (-142.7826, -11.1718) -> (-143.6533, -12.2863) centre (-142.6606, -12.1645) ccw projected
  line L54 (-143.6533, -12.2863) -> (-139.3392, -47.4224) projected
  arc A90 (-139.3392, -47.4224) -> (-138.2247, -48.2931) centre (-138.3466, -47.3005) ccw projected
  line L55 (-138.2247, -48.2931) -> (-119.6234, -46.0091) projected
  arc A91 (-118.5167, -46.828) -> (-119.6234, -46.0091) centre (-119.5015, -47.0016) ccw projected
  line L56 (-118.5167, -46.828) -> (-116.7258, -56.9851) projected
  arc A92 (-116.7258, -56.9851) -> (-115.5673, -57.7963) centre (-115.7409, -56.8114) ccw projected
  line L57 (-115.5673, -57.7963) -> (-95.9163, -54.3313) projected
  arc A93 (-94.7767, -55.0573) -> (-95.9163, -54.3313) centre (-95.7426, -55.3161) ccw projected
  line L58 (-94.7767, -55.0573) -> (-92.2048, -64.6558) projected
  arc A94 (-92.2048, -64.6558) -> (-90.98, -65.363) centre (-91.2388, -64.397) ccw projected
  line L59 (-90.98, -65.363) -> (-72.5182, -60.4162) projected
  arc A95 (-71.3083, -61.0731) -> (-72.5182, -60.4162) centre (-72.2593, -61.3821) ccw projected
  line L60 (-71.3083, -61.0731) -> (-70.3182, -64.1203) projected
  arc A96 (-70.3182, -64.1203) -> (-69.0581, -64.7623) centre (-69.3671, -63.8112) ccw projected
  line L61 (-69.0581, -64.7623) -> (-45.2817, -57.0369) projected
  arc A97 (-45.2817, -57.0369) -> (-44.6397, -55.7769) centre (-45.5908, -56.0858) ccw projected
  line L62 (-44.6397, -55.7769) -> (-45.4122, -53.3992) projected
  arc A98 (-44.7702, -52.1391) -> (-45.4122, -53.3992) centre (-44.4612, -53.0901) ccw projected
  line L63 (-44.7702, -52.1391) -> (-28.6022, -46.8859) projected
  arc A99 (-28.6022, -46.8859) -> (-27.9602, -45.6258) centre (-28.9113, -45.9348) ccw projected
  line L64 (-27.9602, -45.6258) -> (-28.0844, -45.2433) projected
  arc A100 (-27.4917, -44.0008) -> (-28.0844, -45.2433) centre (-27.1334, -44.9343) ccw projected
  line L65 (-27.4917, -44.0008) -> (-9.4036, -37.0574) projected
  arc A101 (-9.4036, -37.0574) -> (-8.8284, -35.7654) centre (-9.762, -36.1238) ccw projected
  line L66 (-8.8284, -35.7654) -> (-11.5745, -28.6116) projected
  arc A102 (-10.6409, -27.2532) -> (-11.5745, -28.6116) centre (-10.641, -28.2531) ccw projected
  line L67 (-10.6409, -27.2532) -> (5.6231, -27.2532) projected
  arc A103 (6.5567, -28.6116) -> (5.6231, -27.2532) centre (5.623, -28.2533) ccw projected
  line L68 (6.5567, -28.6116) -> (3.8105, -35.7654) projected
  arc A104 (3.8105, -35.7654) -> (4.3858, -37.0574) centre (4.744, -36.1239) ccw projected
  line L69 (4.3858, -37.0574) -> (22.4739, -44.0008) projected
  arc A105 (23.0666, -45.2434) -> (22.4739, -44.0008) centre (22.1155, -44.9344) ccw projected
  line L70 (23.0666, -45.2434) -> (22.9423, -45.6258) projected
  arc A106 (22.9423, -45.6258) -> (23.5844, -46.8859) centre (23.8933, -45.9349) ccw projected
  line L71 (23.5844, -46.8859) -> (39.7523, -52.1392) projected
  arc A107 (40.3944, -53.3993) -> (39.7523, -52.1392) centre (39.4433, -53.0903) ccw projected
  line L72 (40.3944, -53.3993) -> (39.6218, -55.7769) projected
  arc A108 (39.6218, -55.7769) -> (40.2638, -57.037) centre (40.5728, -56.086) ccw projected
  line L73 (40.2638, -57.037) -> (64.0403, -64.7624) projected
  arc A109 (64.0403, -64.7624) -> (65.3003, -64.1204) centre (64.3492, -63.8113) ccw projected
  line L74 (65.3003, -64.1204) -> (66.2904, -61.0732) projected
  arc A110 (67.5003, -60.4163) -> (66.2904, -61.0732) centre (67.2415, -61.3823) ccw projected
  line L75 (67.5003, -60.4163) -> (85.9621, -65.3631) projected
  arc A111 (85.9621, -65.3631) -> (87.1869, -64.656) centre (86.2209, -64.3972) ccw projected
  line L76 (87.1869, -64.656) -> (89.7588, -55.0574) projected
  line L77 (-45.529, -56.2761) -> (-69.3053, -64.0015)
  arc A112 (-69.5574, -63.873) -> (-69.3053, -64.0015) centre (-69.3671, -63.8112) ccw
  line L78 (-69.5574, -63.873) -> (-70.5475, -60.8258)
  arc A113 (-70.5475, -60.8258) -> (-72.7252, -59.6434) centre (-72.2593, -61.3821) ccw
  line L79 (-72.7252, -59.6434) -> (-91.187, -64.5902)
  arc A114 (-91.432, -64.4488) -> (-91.187, -64.5902) centre (-91.2388, -64.397) ccw
  line L80 (-91.432, -64.4488) -> (-94.0039, -54.8502)
  arc A115 (-94.0039, -54.8502) -> (-96.0551, -53.5435) centre (-95.7426, -55.3161) ccw
  line L81 (-96.0551, -53.5435) -> (-115.7062, -57.0084)
  arc A116 (-115.938, -56.8462) -> (-115.7062, -57.0084) centre (-115.7409, -56.8114) ccw
  line L82 (-115.938, -56.8462) -> (-117.7289, -46.6891)
  arc A117 (-117.7289, -46.6891) -> (-119.7209, -45.2151) centre (-119.5015, -47.0016) ccw
  line L83 (-119.7209, -45.2151) -> (-138.3222, -47.499)
  arc A118 (-138.5451, -47.3249) -> (-138.3222, -47.499) centre (-138.3466, -47.3005) ccw
  line L84 (-138.5451, -47.3249) -> (-142.8593, -12.1889)
  arc A119 (-142.685, -11.9658) -> (-142.8593, -12.1889) centre (-142.6606, -12.1645) ccw
  line L85 (-142.685, -11.9658) -> (-126.1332, -9.9335)
  arc A120 (-126.1332, -9.9335) -> (-124.58, -7.8345) centre (-126.3526, -8.147) ccw
  line L86 (-124.58, -7.8345) -> (-125.0371, -5.2423)
  arc A121 (-124.8748, -5.0106) -> (-125.0371, -5.2423) centre (-124.8401, -5.2075) ccw
  line L87 (-124.8748, -5.0106) -> (-100.2546, -0.6694)
  arc A122 (-100.0229, -0.8316) -> (-100.2546, -0.6694) centre (-100.2199, -0.8664) ccw
  line L88 (-100.0229, -0.8316) -> (-98.4339, -9.8436)
  arc A123 (-98.4339, -9.8436) -> (-96.1954, -11.2696) centre (-96.6613, -9.531) ccw
  line L89 (-96.1954, -11.2696) -> (-80.7046, -7.1189)
  arc A124 (-80.4595, -7.2604) -> (-80.7046, -7.1189) centre (-80.6528, -7.3122) ccw
  line L90 (-80.4595, -7.2604) -> (-79.7554, -9.888)
  arc A125 (-79.7554, -9.888) -> (-77.4605, -11.1341) centre (-78.0168, -9.4221) ccw
  line L91 (-77.4605, -11.1341) -> (-69.4534, -8.5324)
  arc A126 (-69.4534, -8.5324) -> (-68.2977, -6.2644) centre (-70.0096, -6.8206) ccw
  line L92 (-68.2977, -6.2644) -> (-69.0703, -3.8865)
  arc A127 (-68.942, -3.6347) -> (-69.0703, -3.8865) centre (-68.8803, -3.8248) ccw
  line L93 (-68.942, -3.6347) -> (-53.2165, 1.4748)
  arc A128 (-53.2165, 1.4748) -> (-52.0923, 3.8318) centre (-53.7728, 3.1867) ccw
  line L94 (-52.0923, 3.8318) -> (-52.1383, 3.9517)
  line L95 (-52.1383, 3.9517) -> (-49.5987, 4.9266)
  arc A129 (-49.5987, 4.9266) -> (-48.5506, 7.2175) centre (-50.2437, 6.6069) ccw
  line L96 (-48.5506, 7.2175) -> (-55.6995, 27.0415)
  arc A130 (-55.6053, 27.2859) -> (-55.6995, 27.0415) centre (-55.5114, 27.1093) ccw
  line L97 (-55.6053, 27.2859) -> (-36.6182, 37.3815)
  arc A131 (-36.6182, 37.3815) -> (-36.2422, 37.6483) centre (-37.4628, 38.97) ccw
  line L98 (-36.2422, 37.6483) -> (-19.4649, 53.1425)
  arc A132 (-19.3291, 53.1956) -> (-19.4649, 53.1425) centre (-19.3291, 52.9954) ccw
  line L99 (-19.3291, 53.1956) -> (14.3114, 53.1956)
  arc A133 (14.4471, 53.1425) -> (14.3114, 53.1956) centre (14.3114, 52.9955) ccw
  line L100 (14.4471, 53.1425) -> (31.2243, 37.6484)
  arc A134 (31.2243, 37.6484) -> (31.6006, 37.3813) centre (32.4462, 38.9715) ccw
  line L101 (31.6006, 37.3813) -> (50.5875, 27.2858)
  arc A135 (50.6818, 27.0414) -> (50.5875, 27.2858) centre (50.4936, 27.1092) ccw
  line L102 (50.6818, 27.0414) -> (43.5328, 7.2176)
  arc A136 (43.5328, 7.2176) -> (44.5811, 4.9264) centre (45.2262, 6.6069) ccw
  line L103 (44.5811, 4.9264) -> (46.9338, 4.0233)
  arc A137 (47.0489, 3.7648) -> (46.9338, 4.0233) centre (46.8621, 3.8365) ccw
  line L104 (47.0489, 3.7648) -> (46.3947, 2.0609)
  line L105 (46.3947, 2.0609) -> (63.924, -3.6347)
  arc A138 (64.0525, -3.8869) -> (63.924, -3.6347) centre (63.8622, -3.825) ccw
  line L106 (64.0525, -3.8869) -> (63.28, -6.2643)
  arc A139 (63.28, -6.2643) -> (64.4357, -8.5325) centre (64.9919, -6.8206) ccw
  line L107 (64.4357, -8.5325) -> (72.4427, -11.1342)
  arc A140 (72.4427, -11.1342) -> (74.7377, -9.8881) centre (72.999, -9.4222) ccw
  line L108 (74.7377, -9.8881) -> (75.4418, -7.2605)
  arc A141 (75.6868, -7.119) -> (75.4418, -7.2605) centre (75.635, -7.3122) ccw
  line L109 (75.6868, -7.119) -> (91.1776, -11.2698)
  arc A142 (91.1776, -11.2698) -> (93.4161, -9.8437) centre (91.6435, -9.5312) ccw
  line L110 (93.4161, -9.8437) -> (95.0052, -0.8317)
  arc A143 (95.2368, -0.6696) -> (95.0052, -0.8317) centre (95.2021, -0.8665) ccw
  line L111 (95.2368, -0.6696) -> (119.8571, -5.0108)
  arc A144 (120.0193, -5.2424) -> (119.8571, -5.0108) centre (119.8224, -5.2077) ccw
  line L112 (120.0193, -5.2424) -> (119.5622, -7.8346)
  arc A145 (119.5622, -7.8346) -> (121.1155, -9.9338) centre (121.3349, -8.1472) ccw
  line L113 (121.1155, -9.9338) -> (137.6674, -11.9661)
  arc A146 (137.8415, -12.1889) -> (137.6674, -11.9661) centre (137.6431, -12.1645) ccw
  line L114 (137.8415, -12.1889) -> (133.5273, -47.3251)
  arc A147 (133.3044, -47.4992) -> (133.5273, -47.3251) centre (133.3287, -47.3007) ccw
  line L115 (133.3044, -47.4992) -> (114.7031, -45.2153)
  arc A148 (114.7031, -45.2153) -> (112.711, -46.6893) centre (114.4838, -47.0019) ccw
  line L116 (112.711, -46.6893) -> (110.9201, -56.8465)
  arc A149 (110.6885, -57.0087) -> (110.9201, -56.8465) centre (110.7232, -56.8118) ccw
  line L117 (110.6885, -57.0087) -> (91.0373, -53.5436)
  arc A150 (91.0373, -53.5436) -> (88.9861, -54.8504) centre (90.7247, -55.3162) ccw
  line L118 (88.9861, -54.8504) -> (86.4141, -64.449)
  arc A151 (86.1692, -64.5904) -> (86.4141, -64.449) centre (86.2209, -64.3972) ccw
  line L119 (86.1692, -64.5904) -> (67.7074, -59.6435)
  arc A152 (67.7074, -59.6435) -> (65.5296, -60.826) centre (67.2415, -61.3823) ccw
  line L120 (65.5296, -60.826) -> (64.5395, -63.8731)
  arc A153 (64.2874, -64.0016) -> (64.5395, -63.8731) centre (64.3492, -63.8113) ccw
  line L121 (64.2874, -64.0016) -> (40.511, -56.2762)
  arc A154 (40.3826, -56.0242) -> (40.511, -56.2762) centre (40.5728, -56.086) ccw
  line L122 (40.3826, -56.0242) -> (41.1552, -53.6465)
  arc A155 (41.1552, -53.6465) -> (39.9995, -51.3784) centre (39.4433, -53.0903) ccw
  line L123 (39.9995, -51.3784) -> (23.8315, -46.1251)
  arc A156 (23.7031, -45.8731) -> (23.8315, -46.1251) centre (23.8933, -45.9349) ccw
  line L124 (23.7031, -45.8731) -> (23.8274, -45.4906)
  arc A157 (23.8274, -45.4906) -> (22.7606, -43.2539) centre (22.1155, -44.9344) ccw
  line L125 (22.7606, -43.2539) -> (4.6724, -36.3105)
  arc A158 (4.5574, -36.0522) -> (4.6724, -36.3105) centre (4.744, -36.1239) ccw
  line L126 (4.5574, -36.0522) -> (7.3035, -28.8983)
  arc A159 (7.3035, -28.8983) -> (5.6231, -26.4532) centre (5.623, -28.2533) ccw
  line L127 (5.6231, -26.4532) -> (-10.641, -26.4532)
  arc A160 (-10.641, -26.4532) -> (-12.3214, -28.8982) centre (-10.641, -28.2531) ccw
  line L128 (-12.3214, -28.8982) -> (-9.5753, -36.0522)
  arc A161 (-9.6903, -36.3105) -> (-9.5753, -36.0522) centre (-9.762, -36.1238) ccw
  line L129 (-9.6903, -36.3105) -> (-27.7784, -43.2539)
  arc A162 (-27.7784, -43.2539) -> (-28.8453, -45.4905) centre (-27.1334, -44.9343) ccw
  line L130 (-28.8453, -45.4905) -> (-28.721, -45.8729)
  arc A163 (-28.8495, -46.1251) -> (-28.721, -45.8729) centre (-28.9113, -45.9348) ccw
  line L131 (-28.8495, -46.1251) -> (-45.0175, -51.3783)
  arc A164 (-45.0175, -51.3783) -> (-46.1731, -53.6464) centre (-44.4612, -53.0901) ccw
  line L132 (-46.1731, -53.6464) -> (-45.4005, -56.024)
  arc A165 (-45.529, -56.2761) -> (-45.4005, -56.024) centre (-45.5908, -56.0858) ccw
  arc A166 (-77.3795, -10.2666) -> (-79.0436, -11.5395) centre (-76.4057, -13.2639) ccw projected
  line L133 (-77.7078, -10.3732) -> (-77.3795, -10.2666) projected
  arc A167 (-78.9827, -9.681) -> (-77.7078, -10.3732) centre (-78.0168, -9.4221) ccw projected
  line L134 (-79.6868, -7.0532) -> (-78.9827, -9.681) projected
  arc A168 (-79.6868, -7.0532) -> (-80.9116, -6.3461) centre (-80.6528, -7.3122) ccw projected
  line L135 (-88.5854, -8.4023) -> (-80.9116, -6.3461) projected
  arc A169 (-84.7256, -10.6308) -> (-88.5854, -8.4023) centre (-87.7697, -11.4464) ccw projected
  arc A170 (-84.7256, -10.6308) -> (-79.0436, -11.5395) centre (-81.6815, -9.8151) ccw projected
  circle A171 centre (-81.6815, -9.8151) radius 1.6 projected
  point P0 (0, 0)
  point P1 (73.6714, -11.092)
  point P2 (15.0376, 52.5972)
  point P3 (0.6316, 53.1956)
  point P4 (-5.6492, 53.1956)
  point P5 (-20.0553, 52.5972)
  point P6 (-78.6892, -11.0919)
  point P7 (-86.3516, -8.632)
  point P8 (-141.1064, -26.4648)
  point P9 (-140.2803, -33.1927)
  point P10 (-71.9812, -59.6037)
  point P11 (-63.1542, -62.0029)
  point P12 (-15.1483, -38.4057)
  point P13 (-11.6856, -30.5543)
  point P14 (6.6678, -30.5543)
  point P15 (10.1305, -38.4057)
  point P16 (58.1363, -62.003)
  point P17 (66.9633, -59.6038)
  point P18 (135.2625, -33.193)
  point P19 (136.0886, -26.465)
  point P20 (81.3338, -8.6321)
  dimension "d5" = 0.8
  constraints: 112 end point, 108 point on circle, 54 centre point, 109 other
  measures "d5" distance between parallel lines of L61 L77
extrude "Extrusion3" cut sketch "Sketch3" against normal through all contours A2 A3 L109 A142 L110 A143 L111 A144 L112 A145 L113 A146 L114 A6 A7 A8 A147 L115 A148 L116 A149 L117 A150 L118 A151 L119 A152 A11 A12 A13 L121 A154 L122 A155 L123 A156 L124 A157 L125 A17 A18 A19 L126 A159 L127 A160 L128 A24 A25 A22 L129 A162 L130 A163 L131 A164 L132 A165 L77 A29 A30 A26 A113 L79 A114 L80 A115 L81 A116 L82 A117 L83 A118 L84 A34 A35 A33 A119 L85 A120 L86 A121 L87 A122 L88 A123 L89 A169 A170 A166 A125 L91 A126 L92 A127 L93 A128 L94 L95 A129 L96 A130 L97 A131 L98 A37 A38 A39 L15 A40 L99 A46 L20 A42 A43 A44 L100 A134 L101 A135 L102 A136 L103 A137 L104 L105 A138 L106 A139 L107 A140 A1
fillet "Fillet1" radius 3.175 2 edges at (-5.6088, 0.8, -48.7956) (0.5912, 0.8, -48.7956)